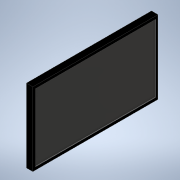
# Autodesk Inventor part: tv1
Saved by Autodesk Inventor 2020 (Build 240168000, 168)
## iProperties
Created: 2021-07-09
Part Number: tv1
Material: Generic
Document SubType Name: Modeling
Designer: pc
Density: 1 g/cm^3
Appearance: Fine Textured - Black
Author: pc
Autodesk Inventor part; units mm, degrees
ref_plane "YZ Plane" through (0, 0, 0) normal (1, 0, 0) x (0, 1, 0)
ref_plane "XZ Plane" through (0, 0, 0) normal (0, 1, 0) x (-1, 0, 0)
ref_plane "XY Plane" through (0, 0, 0) normal (0, 0, 1) x (1, 0, 0)
sketch "Sketch1" plane through (0, 0, 0) normal (1, 0, 0) x (0, 1, 0)
  line L0 (7.7943, 15.2638) -> (-424.0057, 15.2638)
  line L1 (-424.0057, 15.2638) -> (-424.0057, -721.3362)
  line L2 (-424.0057, -721.3362) -> (7.7943, -721.3362)
  line L3 (7.7943, -721.3362) -> (7.7943, 15.2638)
  point P0 (0, 0)
  dimension "d0" = 431.8
  dimension "d1" = 736.6
  constraints: 8 end point, 2 parallel, 1 horizontal, 1 perpendicular
  measures "d0" distance of L2.end L1.end
  measures "d1" distance of L1.end L0.end
extrude "Extrusion1" add sketch "Sketch1" along normal blind 38.1
sketch "Sketch2" plane through (38.1, 0, 0) normal (1, 0, 0) x (0, 0, -1)
  line L0 (0, -9.1095) -> (708.66, -9.1095)
  line L1 (708.66, -9.1095) -> (708.66, -407.8895)
  line L2 (708.66, -407.8895) -> (0, -407.8895)
  line L3 (0, -407.8895) -> (0, -9.1095)
  point P0 (0, 0)
  dimension "d4" = 708.66
  dimension "d5" = 398.78
  constraints: 8 end point, 2 parallel, 1 horizontal, 1 perpendicular
  measures "d4" distance of L1.end L2.end
  measures "d5" distance of L0.end L1.end
extrude "Extrusion2" cut sketch "Sketch2" against normal blind 5.08
sketch "Sketch3" plane through (0, 0, 0) normal (-1, 0, 0) x (0, 0, 1)
  line L0 (-470.803, -170.5411) -> (-267.603, -170.5411)
  line L1 (-267.603, -170.5411) -> (-267.603, -246.7411)
  line L2 (-267.603, -246.7411) -> (-470.803, -246.7411)
  line L3 (-470.803, -246.7411) -> (-470.803, -170.5411)
  point P0 (0, 0)
  constraints: 8 end point, 2 parallel, 1 horizontal, 1 perpendicular
extrude "Extrusion3" add sketch "Sketch3" along normal blind 10.16
sketch "Sketch4" plane through (-10.16, 0, 0) normal (-1, 0, 0) x (0, 0, 1)
  line L0 (-508, -138.5372) -> (-232.9195, -138.5372)
  line L1 (-232.9195, -138.5372) -> (-232.9195, -283.012)
  line L2 (-232.9195, -283.012) -> (-508, -283.012)
  line L3 (-508, -283.012) -> (-508, -138.5372)
  point P0 (0, 0)
  constraints: 8 end point, 2 parallel, 1 horizontal, 1 perpendicular
extrude "Extrusion4" add sketch "Sketch4" along normal blind 15.24
body "Solid1"
